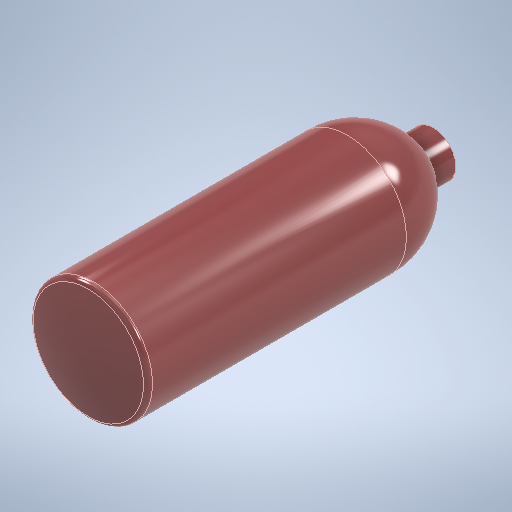
# Autodesk Inventor part: tank
Saved by Autodesk Inventor 2026.1 (Build 301233020, 233B)
## iProperties
Created: 2026-01-22
Part Number: tank
Material: Generic
Document SubType Name: Modeling
Designer: user
Density: 1 g/cm^3
Appearance: Chestnut
Author: user
Autodesk Inventor part; units mm, degrees
ref_plane "YZ Plane" through (0, 0, 0) normal (1, 0, 0) x (0, 1, 0)
ref_plane "XZ Plane" through (0, 0, 0) normal (0, 1, 0) x (-1, 0, 0)
ref_plane "XY Plane" through (0, 0, 0) normal (0, 0, 1) x (1, 0, 0)
sketch "Sketch1" plane through (0, 0, 0) normal (0, 0, 1) x (1, 0, 0)
  circle A0 centre (0, 0) radius 55
  circle A1 centre (0, 0) radius 50
  dimension "d0" = 110
  dimension "d1" = 100
  constraints: 2 centre point, 2 coincident
  measures "d0" diameter of A0
  measures "d1" diameter of A1
extrude "Extrusion1" add sketch "Sketch1" along normal blind 220
sketch "Sketch2" plane through (0, 0, 0) normal (0, 1, 0) x (-1, 0, 0)
  line L0 (55, 0) -> (-55, 0) projected
  line L1 (0, 0) -> (55, 0)
  line L2 (0, 0) -> (0, -60)
  line L3 (0, -60) -> (21, -60)
  arc A0 (21, -60) -> (55, 0) centre (-11.9561, -1.6915) ccw
  line L4 (0, 0) -> (50, 0)
  line L5 (0, -60) -> (0, -55)
  line L6 (0, -55) -> (18, -55)
  arc A1 (21, -55) -> (50, 0) centre (-15.1736, -0.7812) ccw
  line L7 (18, -55) -> (21, -55)
  dimension "d4" = 60
  dimension "d5" = 21
  dimension "d6" = 50
  dimension "d7" = 5
  dimension "d8" = 18
  constraints: 14 end point, 4 point on circle, 3 perpendicular, 2 centre point, 2 point on line, 1 collinear, 1 horizontal
  measures "d4" distance of L1.start L2.end
  measures "d5" distance of L2.end L3.end
  measures "d6" distance of L1.start L4.end
  measures "d7" distance of L2.end L5.end
  measures "d8" distance of L5.end L6.end
revolve "Revolution1" add sketch "Sketch2" angle 360 about axis through (0, 0, 0) along (0, 0, -1) contours A0 L3 L2 L6 L7 A1 L0
sketch "Sketch3" plane through (0, 0, -60) normal (0, 0, -1) x (-1, 0, 0)
  circle A0 centre (0, 0) radius 21
  circle A1 centre (0, 0) radius 16
  dimension "d10" = 32
  constraints: 2 centre point, 2 coincident
  measures "d10" diameter of A1
extrude "Extrusion2" add sketch "Sketch3" along normal blind 20
sketch "Sketch4" plane through (0, 0, -60) normal (0, 0, -1) x (-1, 0, 0)
  circle A0 centre (0, 0) radius 16
  constraints: 1 centre point, 1 coincident
extrude "Extrusion3" cut sketch "Sketch4" against normal blind 20
sketch "Sketch5" plane through (0, 0, 0) normal (0, 1, 0) x (-1, 0, 0)
  line L0 (55, 220) -> (-55, 220) projected
  line L1 (0, 220) -> (55, 220)
  line L2 (55, 0) -> (55, 220) projected
  line L3 (55, 220) -> (55, 240)
  line L4 (0, 220) -> (0, 250)
  arc A0 (55, 240) -> (0, 250) centre (-11.131, 32.5294) ccw
  line L5 (55, 220) -> (50, 220)
  line L6 (50, 220) -> (50, 235)
  line L7 (0, 220) -> (5, 220)
  line L8 (0, 250) -> (0, 245)
  arc A1 (50, 235) -> (0, 245) centre (-19.5494, 17.2528) ccw
  point P0 (0, 0)
  dimension "d15" = 20
  dimension "d16" = 30
  dimension "d17" = 5
  dimension "d18" = 15
  dimension "d19" = 5
  dimension "d20" = 5
  constraints: 14 end point, 4 point on circle, 4 point on line, 2 centre point, 2 vertical, 1 horizontal, 1 midpoint, 1 perpendicular
  measures "d15" distance of L2.end L3.end
  measures "d16" distance of L1.start L4.end
  measures "d17" distance of L2.end L5.end
  measures "d18" distance of L5.end L6.end
  measures "d19" distance of L1.start L7.end
  measures "d20" distance of L4.end L8.end
revolve "Revolution2" add sketch "Sketch5" angle 360 about axis through (0, 0, 220) along (0, 0, 1) contours L0 L6 A1 L4 A0 L3
fillet "Fillet1" radius 5 1 edges at (55, 0, 240)
body "Solid1"
